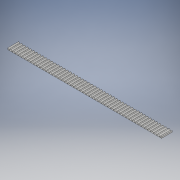
# Autodesk Inventor part: belt new
Saved by Autodesk Inventor 2019 (Build 230136000, 136)
## iProperties
Created: 2020-02-11
Part Number: belt new
Material: Generic
Document SubType Name: Modeling
Designer: Vinayak
Density: 1 g/cm^3
Appearance: Default
Author: Vinayak
Autodesk Inventor part; units mm, degrees
ref_plane "YZ Plane" through (0, 0, 0) normal (1, 0, 0) x (0, 1, 0)
ref_plane "XZ Plane" through (0, 0, 0) normal (0, 1, 0) x (-1, 0, 0)
ref_plane "XY Plane" through (0, 0, 0) normal (0, 0, 1) x (1, 0, 0)
sketch "Sketch1" plane through (0, 0, 0) normal (0, 0, 1) x (1, 0, 0)
  line L0 (0, 0.2) -> (0, 0)
  arc A0 (0, 0.6761) -> (-0.4761, 0.2) centre (0, 0.2) ccw
  line L1 (-0.4761, 0.2) -> (-0.9521, 0.2)
  line L2 (-1.4281, 0) -> (-1.4281, 0.676)
  arc A1 (-0.9521, 0.2) -> (-1.4281, 0.676) centre (-1.4281, 0.2) ccw
  line L3 (-1.9046, 0.2) -> (-1.9041, 0.2)
  line L4 (0, 0) -> (-1.4281, 0)
  line L5 (0, 0.2) -> (0, 0.6761)
  line L6 (-0.9521, 0.2) -> (-0.4761, 0.2)
  line L7 (0, 0) -> (0, 0.6761)
  line L8 (-1.4281, 0) -> (-1.4281, 0.676)
  dimension "d0" = 1.9046
  dimension "d2" = 0.9522
  constraints: 18 end point, 4 point on circle, 2 centre point, 2 vertical, 1 coincident, 1 collinear, 1 horizontal, 1 parallel
  measures "d0" distance of L3.start L0.start
  measures "d2" diameter of A0
extrude "Extrusion1" add sketch "Sketch1" along normal blind 5
pattern_linear "Rectangular Pattern1" count 50 spacing 1.4279 along (1, 0, 0)
body "Solid1"
